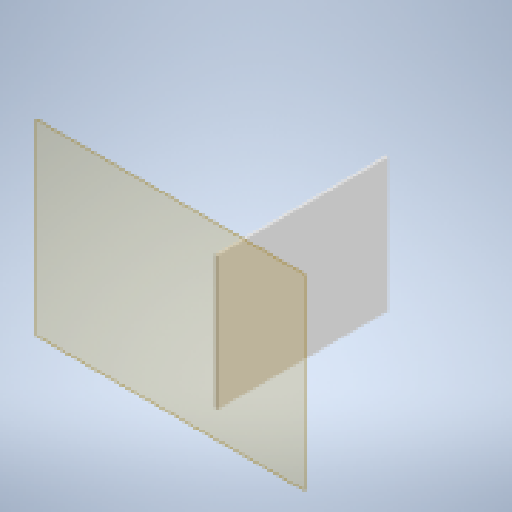
# Autodesk Inventor part: Baffle
Saved by Autodesk Inventor 2023 (Build 270158000, 158)
## iProperties
Created: 2022-08-07
Part Number: Baffle
Material: Generic
Document SubType Name: Modeling
Designer: techv
Density: 1 g/cm^3
Appearance: Default
Author: techv
Autodesk Inventor part; units mm, degrees
ref_plane "YZ Plane" through (0, 0, 0) normal (1, 0, 0) x (0, 1, 0)
ref_plane "XZ Plane" through (0, 0, 0) normal (0, 1, 0) x (-1, 0, 0)
ref_plane "Work Plane1" through (0, 0, 0) normal (0, 0, 1) x (1, 0, 0)
sketch "Sketch1" plane through (0, 0, 0) normal (0, 0, 1) x (1, 0, 0)
  line L0 (-93, 209) -> (-93, 3) projected
  line L1 (-93, 209) -> (-96, 209)
  line L2 (-96, 209) -> (-96, 3)
  line L3 (-96, 3) -> (-93, 3)
  line L4 (-93, 3) -> (-93, 209)
  line L5 (-93, 209) -> (-93, 106)
  line L6 (-93, 106) -> (-94.5, 106)
  line L7 (-93, 189) -> (-96, 189)
  line L8 (-96, 189) -> (-96, 23)
  line L9 (-96, 23) -> (-93, 23)
  line L10 (-93, 23) -> (-93, 189)
  line L11 (-93, 189) -> (-96, 23) construction
  line L12 (-96, 189) -> (-93, 23) construction
  point P0 (0, 0)
  dimension "d0" = 3
  dimension "d1" = 103
  dimension "d2" = 1.5
  dimension "d3" = 166
  constraints: 24 end point, 4 parallel, 3 midpoint, 3 perpendicular, 2 horizontal, 1 point on line
  measures "d0" distance of L3.end L2.end
  measures "d1" distance of L0.start L5.end
  measures "d2" distance of L5.end L6.end
  measures "d3" distance of L8.end L7.end
ref_plane "Work Plane2" through (-303, 0, -212) normal (0, 0, -1) x (0, 1, 0)
extrude "Extrusion1" add sketch "Sketch1" against normal up to surface (212 mm away) contours L0 L9 L2 L7
body "Solid1"
